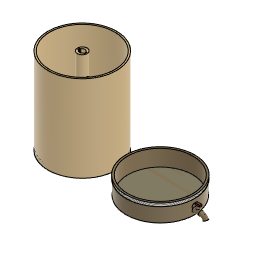
Composting Bin v2 (1) (Autodesk Fusion 360 design; units mm, degrees)
Autodesk Fusion 360 part; units mm, degrees
sketch "Sketch1" plane through (0, 0, 0) normal (0, 0, 1) x (1, 0, 0)
  circle A0 centre (0, 0) radius 525
  circle A1 centre (0, 0) radius 500
  dimension "d1" = 1000
  dimension "d2" = 1050
  constraint coincident A0.centre A1.centre
  measures "d1" diameter of A1
  measures "d2" diameter of A0
extrude "Extrude1" add sketch "Sketch1" along normal blind 1000 makes body 1
extrude "Extrude2" add 1 faces at (512.8505, -50.9228, 1000) along direction (0, 0, 1) blind 300 on bodies 1 bodies 1
sketch "Sketch2" plane through (0, 0, 0) normal (0, 0, 1) x (1, 0, 0)
  circle A0 centre (0, 0) radius 525
  circle A1 centre (0, 0) radius 75
  dimension "d7" = 1050
  dimension "d8" = 150
  constraint coincident A0.centre A1.centre
  measures "d7" diameter of A0
  measures "d8" diameter of A1
extrude "Extrude3" add sketch "Sketch2" along normal blind 1300 separate body contours A1 makes body 2
sketch "Sketch3" plane through (0, 0, 0) normal (0, 0, 1) x (1, 0, 0)
  circle A0 centre (0, 0) radius 525
  dimension "d11" = 1050
  constraint coincident A0.centre origin
  measures "d11" diameter of A0
extrude "Extrude4" add sketch "Sketch3" against normal blind 25 bodies 1 2
extrude "Extrude5" add 1 faces at (18.6055, 20.7304, 1300) along direction (0, 0, -1) blind 1350 on bodies 1 bodies 1
sketch "Sketch4" plane through (0, 0, -50) normal (0, 0, -1) x (1, 0, 0)
  circle A0 centre (0, 0) radius 75
  line L0 (54.9993, -15.7564) -> (-54.9993, -15.7564)
  line L1 (-54.9993, -15.7564) -> (-54.9993, 15.7564)
  line L2 (-54.9993, 15.7564) -> (54.9993, 15.7564)
  line L3 (54.9993, 15.7564) -> (54.9993, -15.7564)
  line L4 (54.9993, -15.7564) -> (-54.9993, 15.7564) construction
  line L5 (-54.9993, -15.7564) -> (54.9993, 15.7564) construction
  arc A1 (39.9527, 11.4457) -> (-39.9527, 11.4457) centre (0, 0) ccw
  arc A2 (-39.9527, -11.4457) -> (39.9527, -11.4457) centre (0, 0) ccw
  constraint coincident A0.centre A1.centre
  constraint horizontal L0
  constraint perpendicular L0 L1
  constraint parallel L0 L2
  constraint parallel L1 L3
  constraint coincident L4 A0.centre
  constraint coincident L5 A0.centre
  constraint coincident L4 A2.end
  constraint coincident L5 A1.start
  constraint coincident L4 A1.end
  constraint coincident L5 A2.start
  constraint concentric A1 A2
extrude "Extrude6" cut sketch "Sketch4" against normal blind 1500 contours L0 L1 L2 L3 | L0 A2 | L2 A1 bodies 1
sketch "Sketch5" plane through (0, 0, -25) normal (0, 0, -1) x (1, 0, 0)
  circle A0 centre (0, 0) radius 75
  circle A1 centre (0, 0) radius 525
  circle A2 centre (0, 150) radius 25
  circle A3 centre (0, 250) radius 25
  circle A4 centre (0, 350) radius 25
  circle A5 centre (0, 450) radius 25
  circle A6 centre (0, -148.3454) radius 25
  circle A7 centre (0, -348.3454) radius 25
  circle A8 centre (0, -248.3454) radius 25
  circle A9 centre (0, -448.3454) radius 25
  circle A10 centre (148.3454, 0) radius 25
  circle A11 centre (248.3454, 0) radius 25
  circle A12 centre (348.3454, 0) radius 25
  circle A13 centre (448.3454, 0) radius 25
  circle A14 centre (-150, 0) radius 25
  circle A15 centre (-250, 0) radius 25
  circle A16 centre (-350, 0) radius 25
  circle A17 centre (-450, 0) radius 25
  circle A18 centre (-102.0712, 102.2193) radius 25
  circle A19 centre (-185.481, 185.75) radius 25
  circle A20 centre (-271.6071, 272.0011) radius 25
  circle A21 centre (-327.7733, 328.2487) radius 25
  circle A22 centre (102.0712, 102.2193) radius 25
  circle A23 centre (185.481, 185.75) radius 25
  circle A24 centre (271.6071, 272.0011) radius 25
  circle A25 centre (327.7733, 328.2487) radius 25
  circle A26 centre (-102.0712, -102.2193) radius 25
  circle A27 centre (-185.481, -185.75) radius 25
  circle A28 centre (-271.6071, -272.0011) radius 25
  circle A29 centre (-327.7733, -328.2487) radius 25
  circle A30 centre (102.0712, -102.2193) radius 25
  circle A31 centre (185.481, -185.75) radius 25
  circle A32 centre (271.6071, -272.0011) radius 25
  circle A33 centre (327.7733, -328.2487) radius 25
  point P0 (310.1084, 310.5582)
  point P1 (310.1084, -310.5582)
  dimension "d18" = 50
  dimension "d19" = 50
  dimension "d20" = 50
  dimension "d21" = 50
  dimension "d22" = 50
  dimension "d23" = 50
  dimension "d24" = 50
  dimension "d25" = 50
  measures "d18" diameter of A2
  measures "d19" diameter of A3
  measures "d20" diameter of A4
  measures "d21" diameter of A5
  measures "d22" diameter of A18
  measures "d23" diameter of A19
  measures "d24" diameter of A20
  measures "d25" diameter of A21
extrude "Extrude7" cut sketch "Sketch5" against normal blind 50 contours A2 | A3 | A4 | A5 | A6 | A7 | A8 | A9 | A10 | A11 | A12 | A13 | A14 | A15 | A16 | A17 | A18 | A19 | A20 | A21 | A22 | A23 | A24 | A25 | A26 | A27 | A28 | A29 | A30 | A31 | A32 | A33 bodies 1
sketch "Sketch6" plane through (0, 0, 0) normal (0, 0, 1) x (1, 0, 0)
  circle A0 centre (1200, 0) radius 525
  circle A1 centre (1200, 0) radius 500
  dimension "d28" = 1050
  dimension "d29" = 1000
  constraint concentric A0 A1
  measures "d28" diameter of A0
  measures "d29" diameter of A1
extrude "Extrude8" add sketch "Sketch6" along normal blind 200 separate body makes body 3
sketch "Sketch7" plane through (0, 0, 0) normal (0, 0, -1) x (1, 0, 0)
  circle A0 centre (1200, 0) radius 500
  circle A1 centre (1200, 0) radius 525
  circle A2 centre (1200, 0) radius 525
  constraint concentric A0 A2
extrude "Extrude9" add sketch "Sketch7" along normal blind 20 contours A0 | A1 A2 bodies 3
sketch "Sketch8" plane through (0, 0, 200) normal (0, 0, 1) x (-1, 0, 0)
  circle A0 centre (-1200, 0) radius 500
  circle A1 centre (-1200, 0) radius 525
  circle A2 centre (-1200, 0) radius 512.5
  circle A3 centre (-1200, 0) radius 500
  dimension "d34" = 1025
  dimension "d35" = 1000
  constraint concentric A0 A2
  constraint concentric A2 A3
  measures "d34" diameter of A2
  measures "d35" diameter of A3
extrude "Extrude10" add sketch "Sketch8" along normal blind 50 contours A2 bodies 3
sketch "Sketch9" plane through (0, 0, 0) normal (0, 0, 1) x (-1, 0, 0)
  circle A0 centre (-1200, 0) radius 500
sketch "Sketch10" plane through (0, 0, 0) normal (1, 0, 0) x (0, 1, 0)
ref_plane "WorkPlane1" through (1800, 0, 0) normal (1, 0, 0) x (0, 1, 0)
sketch "Sketch11" plane through (1800, 0, 0) normal (1, 0, 0) x (0, 1, 0)
  circle A0 centre (0, 100) radius 33.5903
extrude "Extrude11" cut sketch "Sketch11" against normal blind 200 bodies 3
thread "Thread1" "ISO Metric profile 1060.0 M1060x8 6g" major diameter 1059.545 minor diameter 1050.2952 pitch 8 angle 60 resizes the face on face at (690.0467, 51.0285, 216.6667) on bodies 3
sketch "Sketch12" plane through (0, 0, -25) normal (0, 0, -1) x (1, 0, 0)
  circle A0 centre (-185.481, -185.75) radius 25
  circle A1 centre (-327.7733, 328.2487) radius 25
  circle A2 centre (-150, 0) radius 25
  circle A3 centre (0, -348.3454) radius 25
  circle A4 centre (185.481, -185.75) radius 25
  circle A5 centre (348.3454, 0) radius 25
  circle A6 centre (185.481, 185.75) radius 25
  circle A7 centre (0, 350) radius 25
  circle A8 centre (0, 250) radius 25
  circle A9 centre (271.6071, 272.0011) radius 25
  circle A10 centre (248.3454, 0) radius 25
  circle A11 centre (271.6071, -272.0011) radius 25
  circle A12 centre (0, -248.3454) radius 25
  circle A13 centre (-102.0712, 102.2193) radius 25
  circle A14 centre (-450, 0) radius 25
  circle A15 centre (-271.6071, -272.0011) radius 25
  circle A16 centre (-250, 0) radius 25
  circle A17 centre (-271.6071, 272.0011) radius 25
  circle A18 centre (-102.0712, -102.2193) radius 25
  circle A19 centre (0, -448.3454) radius 25
  circle A20 centre (102.0712, -102.2193) radius 25
  circle A21 centre (448.3454, 0) radius 25
  circle A22 centre (102.0712, 102.2193) radius 25
  circle A23 centre (0, 450) radius 25
  circle A24 centre (0, 150) radius 25
  circle A25 centre (327.7733, 328.2487) radius 25
  circle A26 centre (148.3454, 0) radius 25
  circle A27 centre (327.7733, -328.2487) radius 25
  circle A28 centre (0, -148.3454) radius 25
  circle A29 centre (-185.481, 185.75) radius 25
  circle A30 centre (-350, 0) radius 25
  circle A31 centre (-327.7733, -328.2487) radius 25
  circle A32 centre (0, 0) radius 75
  circle A33 centre (0, 0) radius 525
  circle A34 centre (0, 0) radius 500
  circle A35 centre (0, 0) radius 512.5
  dimension "d43" = 1000
  dimension "d44" = 1025
  constraint concentric A32 A34
  constraint concentric A34 A35
  measures "d43" diameter of A34
  measures "d44" diameter of A35
extrude "Extrude12" cut sketch "Sketch12" against normal blind 50 contours A35 bodies 1 makes body 4 at (522.3912, -52.2731, 433.3333)
extrude "Extrude13" add 1 faces at (-152.8739, 366.6221, 0) along direction (0, 0, 1) blind 10 on bodies 1 bodies 1
extrude "Extrude14" add 1 faces at (-152.8739, 366.6221, 10) along direction (0, 0, 1) blind 20 on bodies 1 bodies 1 4
sketch "Sketch13" plane through (0, 0, 0) normal (1, 0, 0) x (0, 1, 0)
ref_plane "WorkPlane2" through (1700, 0, 0) normal (1, 0, 0) x (0, 1, 0)
sketch "Sketch14" plane through (1700, 0, 0) normal (1, 0, 0) x (0, 1, 0)
  circle A0 centre (0, 100) radius 35
  dimension "d52" = 70
  measures "d52" diameter of A0
sketch "Sketch15" plane through (0, 0, 0) normal (0, 1, 0) x (1, 0, 0)
  line L0 (1700, -100) -> (1822.0165, -100)
  arc A0 (1822.0165, -100) -> (1900, -50) centre (1822.0165, -14.1857) ccw
  constraint horizontal L0
  constraint tangent L0 A0
sketch "Sketch16" plane through (1700, 0, 0) normal (1, 0, 0) x (0, 1, 0)
sketch "Sketch17" plane through (1700, 0, 0) normal (1, 0, 0) x (0, 1, 0)
  circle A0 centre (0, 100) radius 25
  dimension "d53" = 50
  measures "d53" diameter of A0
sweep "Sweep1" add profiles "Sketch14" path "Sketch15" along L0 A0 section 1 separate body makes body 5
hole "Hole1" at (1700, 0, 100) direction (1, 0, 0) diameter 40 depth 70 tip angle 118 bodies 5
hole "Hole2" at (1899.4037, -0.1086, 49.7262) direction (-0.417347, 0, 0.908747) diameter 40 depth 40 tip angle 118 bodies 5
ref_plane "WorkPlane3" through (1788.2768, 0, 135) normal (0, 0, 1) x (0, 1, 0)
sketch "Sketch18" plane through (0, 0, 135) normal (0, 0, 1) x (1, 0, 0)
  circle A0 centre (1775, 0) radius 18.0579
extrude "Extrude15" add sketch "Sketch18" along normal mid plane 100 bodies 5
sketch "Sketch19" plane through (0, 0, 185) normal (0, 0, 1) x (-1, 0, 0)
  circle A0 centre (-1775, 0) radius 18.0579
  line L0 (-1747.7824, -16.2807) -> (-1822.4821, -16.2807)
  line L1 (-1822.4821, -16.2807) -> (-1822.4821, 15.323)
  line L2 (-1822.4821, 15.323) -> (-1747.7824, 15.323)
  line L3 (-1747.7824, 15.323) -> (-1747.7824, -16.2807)
  constraint horizontal L0
  constraint vertical L1
  constraint horizontal L2
  constraint vertical L3
extrude "Extrude16" add sketch "Sketch19" along normal blind 25 separate body contours A0 L0 L2 | A0 L0 L2 L3 | A0 L0 L1 L2 makes body 6
ref_plane "WorkPlane4" through (75, 0, 1181.149) normal (1, 0, 0) x (0, -1, 0)
sketch "Sketch20" plane through (75, 0, 0) normal (1, 0, 0) x (0, 1, 0)
  line L0 (0, 400) -> (-24.1819, 400)
  line L1 (-24.1819, 400) -> (-24.1819, 795.0557)
  line L2 (-24.1819, 795.0557) -> (0, 795.0557)
  line L3 (0, 795.0557) -> (0, 400)
  constraint horizontal L0
  constraint vertical L1
  constraint horizontal L2
  constraint vertical L3
extrude "Extrude17" add sketch "Sketch20" along normal blind 400 separate body makes body 7
sketch "Sketch21" plane through (0, 0, 0) normal (0, 1, 0) x (-1, 0, 0)
  line L0 (-75, 400) -> (-75, 795.0557)
  line L1 (-75, 795.0557) -> (-475, 795.0557)
  line L2 (-475, 795.0557) -> (-475, 400)
  line L3 (-475, 400) -> (-75, 400)
  line L4 (-105.194, 677.2693) -> (-238.5391, 677.2693)
  line L5 (-238.5391, 677.2693) -> (-238.5391, 597.5279)
  line L6 (-238.5391, 597.5279) -> (-105.194, 597.5279)
  line L7 (-105.194, 597.5279) -> (-105.194, 677.2693)
  line L8 (-266.6866, 597.5279) -> (-398.5483, 597.5279)
  line L9 (-398.5483, 597.5279) -> (-398.5483, 675.6061)
  line L10 (-398.5483, 675.6061) -> (-266.6866, 675.6061)
  line L11 (-266.6866, 675.6061) -> (-266.6866, 597.5279)
  line L12 (-105.194, 537.818) -> (-398.5483, 537.818)
  line L13 (-398.5483, 537.818) -> (-398.5483, 490.407)
  line L14 (-398.5483, 490.407) -> (-105.194, 490.407)
  line L15 (-105.194, 490.407) -> (-105.194, 537.818)
  constraint horizontal L4
  constraint vertical L5
  constraint horizontal L6
  constraint vertical L7
  constraint horizontal L8
  constraint vertical L9
  constraint horizontal L10
  constraint vertical L11
  constraint horizontal L12
  constraint vertical L13
  constraint horizontal L14
  constraint vertical L15
extrude "Extrude18" cut sketch "Sketch21" against normal blind 50 contours L4 L5 L6 L7 | L8 L9 L10 L11 | L12 L13 L14 L15 bodies 7
mirror "Mirror1" about plane through (0, 0, 0) normal (1, 0, 0) of bodies 7 makes body 8
move_body "Move1" bodies 7 to x (1, 0, 0) y (0, 1, 0) z (0, 0, 1) at (0, 10, 0)
move_body "Move2" bodies 8 to x (1, 0, 0) y (0, 1, 0) z (0, 0, 1) at (0, 10, 0)
move_body "Move3" bodies 8 to x (1, 0, 0) y (0, 1, 0) z (0, 0, 1) at (0, 0, -100)
move_body "Move4" bodies 7 to x (1, 0, 0) y (0, 1, 0) z (0, 0, 1) at (0, 0, 100)
move_body "Move5" bodies 7 to x (1, 0, 0) y (0, 1, 0) z (0, 0, 1) at (0, 0, 100)
move_body "Move6" bodies 8 to x (1, 0, 0) y (0, 1, 0) z (0, 0, 1) at (0, 0, -100)
move_body "Move7" bodies 5 to x (1, 0, 0) y (0, 1, 0) z (0, 0, 1) at (0, 0, -50)
move_body "Move8" bodies 6 to x (1, 0, 0) y (0, 1, 0) z (0, 0, 1) at (0, 0, -50)
ref_plane "WorkPlane5" through (1725, 0, 90.1468) normal (1, 0, 0) x (0, -1, 0)
sketch "Sketch22" plane through (1725, 0, 0) normal (1, 0, 0) x (0, 1, 0)
  circle A0 centre (0, 100) radius 35.3553
extrude "Extrude19" add sketch "Sketch22" against normal blind 25 bodies 3 6 5
sketch "Sketch23" plane through (1725, 0, 0) normal (1, 0, 0) x (0, 1, 0)
  arc A0 (24.7475, 74.75) -> (-24.7475, 74.75) centre (0, 50) ccw
  arc A1 (24.7475, 74.75) -> (0, 135.3553) centre (0, 100) ccw
  arc A2 (0, 135.3553) -> (-24.7475, 74.75) centre (0, 100) ccw
  circle A3 centre (0, 50) radius 35
  circle A4 centre (0, 50) radius 35
  constraint concentric A0 A3
  constraint coincident A0.end A3
  constraint concentric A3 A4
extrude "Extrude20" cut sketch "Sketch23" against normal blind 150 contours A0 A3 A4 bodies 3
extrude "Extrude21" add 1 faces at (1725, -22.8318, 69.3569) along direction (-1, 0, 0) blind 25 on bodies 3 bodies 3
hole "Hole3" at (1700, 0, 50) direction (1, 0, 0) diameter 30 depth 180 tip angle 118 bodies 3
